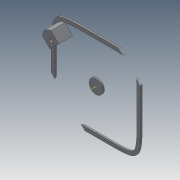
# Autodesk Inventor part: Part1
Saved by Autodesk Inventor 2014 SP1 (Build 180222100, 222)
## iProperties
Created: 2014-04-02
Part Number: Part1
Material: Generic
Document SubType Name: Modeling
Designer: tom
Density: 1 g/cm^3
Appearance: Default
Author: tom
Autodesk Inventor part; units mm, degrees
ref_plane "YZ Plane" through (0, 0, 0) normal (1, 0, 0) x (0, 1, 0)
ref_plane "XZ Plane" through (0, 0, 0) normal (0, 1, 0) x (-1, 0, 0)
ref_plane "XY Plane" through (0, 0, 0) normal (0, 0, 1) x (1, 0, 0)
sketch "Sketch1" plane through (0, 0, 0) normal (0, 0, 1) x (1, 0, 0)
  line L0 (-82.2587, 0) -> (-82.2587, 66.0349) construction
  line L1 (-82.2587, 66.0349) -> (-82.5436, 82.5437) construction
  line L2 (-82.5436, 82.5437) -> (-65.75, 82.0022) construction
  line L3 (-65.75, 82.0022) -> (0.29, 81.9737) construction
  spline S0 degree 4 poles (-82.2587, 0) (-82.2587, 66.0349) (-82.5436, 82.5437) (-65.75, 82.0022) (0.29, 81.9737) knots 1 1 1 1 1 2 2 2 2 2
  spline S1 degree 4 poles (-0.0001, -80.2641) (-66.0349, -80.2631) (-82.5436, -82.5437) (-82.2587, -66.0349) (-82.2587, 0) knots 1 1 1 1 1 2 2 2 2 2
  line L4 (-0.0001, -80.2641) -> (-66.0349, -80.2631) construction
  line L5 (-66.0349, -80.2631) -> (-82.5436, -82.5437) construction
  line L6 (-82.5436, -82.5437) -> (-82.2587, -66.0349) construction
  line L7 (-82.2587, -66.0349) -> (-82.2587, 0) construction
  spline S2 degree 4 poles (81.9738, 0.0005) (81.9826, -66.0349) (82.5437, -82.5436) (66.0349, -80.2652) (-0.0001, -80.2641) knots 1 1 1 1 1 2 2 2 2 2
  line L8 (81.9738, 0.0005) -> (81.9826, -66.0349) construction
  line L9 (81.9826, -66.0349) -> (82.5437, -82.5436) construction
  line L10 (82.5437, -82.5436) -> (66.0349, -80.2652) construction
  line L11 (66.0349, -80.2652) -> (-0.0001, -80.2641) construction
  spline S3 degree 4 poles (0.29, 81.9737) (66.0431, 81.9454) (82.5436, 82.5436) (81.9649, 66.0349) (81.9738, 0.0005) knots 1 1 1 1 1 2 2 2 2 2
  line L12 (0.29, 81.9737) -> (66.0431, 81.9454) construction
  line L13 (66.0431, 81.9454) -> (82.5436, 82.5436) construction
  line L14 (82.5436, 82.5436) -> (81.9649, 66.0349) construction
  line L15 (81.9649, 66.0349) -> (81.9738, 0.0005) construction
  circle A0 centre (0, 0) radius 12.7
  spline S4 degree 5 poles (75.1158, -0.0005) (75.1151, 4.7038) (75.1174, 9.4081) (75.1176, 14.1124) (75.1034, 22.44) (75.0077, 30.7672) (74.9416, 34.3899) (74.7649, 40.6623) (74.3822, 46.9251) (74.1686, 49.5676) (73.6967, 53.9768) (72.8746, 58.3337) (72.4687, 60.0672) (71.6353, 62.8858) (70.347, 65.5172) (69.7572, 66.5071) (68.3459, 68.3278) (66.529, 69.744) (65.543, 70.3346) (62.923, 71.6236) (60.1151, 72.4579) (58.3888, 72.8639) (54.0494, 73.6867) (49.6575, 74.1591) (47.0251, 74.3729) (40.7867, 74.7564) (34.5385, 74.934) (30.9299, 75.0006) (22.6362, 75.0978) (14.342, 75.1137) (9.657, 75.1147) (4.972, 75.1137) (0.287, 75.1157) knots 0 0 0 0 0 0 0.169519 0.169519 0.169519 0.300085 0.300085 0.300085 0.395596 0.395596 0.395596 0.459735 0.459735 0.459735 0.500964 0.500964 0.500964 0.542086 0.542086 0.542086 0.605973 0.605973 0.605973 0.701119 0.701119 0.701119 0.831177 0.831177 0.831177 1 1 1 1 1 1
  spline S5 degree 5 poles (0.287, 75.1157) (-4.4205, 75.1178) (-9.1281, 75.1224) (-13.8357, 75.1248) (-22.1755, 75.114) (-30.5149, 75.0207) (-34.1464, 74.9554) (-40.4414, 74.7792) (-46.7267, 74.3962) (-49.3828, 74.1821) (-53.824, 73.7076) (-58.2129, 72.8821) (-59.9648, 72.4734) (-62.8221, 71.6316) (-65.4927, 70.333) (-66.5029, 69.7357) (-68.3594, 68.3111) (-69.8124, 66.4769) (-70.4194, 65.4828) (-71.7396, 62.8516) (-72.6013, 60.027) (-73.0204, 58.2951) (-73.8722, 53.9442) (-74.3672, 49.5377) (-74.5926, 46.898) (-74.9998, 40.6409) (-75.1937, 34.3731) (-75.2678, 30.7528) (-75.3783, 22.4301) (-75.4, 14.1068) (-75.4022, 9.4045) (-75.4007, 4.7023) (-75.4007, 0) knots 0 0 0 0 0 0 0.168867 0.168867 0.168867 0.299158 0.299158 0.299158 0.394725 0.394725 0.394725 0.459234 0.459234 0.459234 0.50104 0.50104 0.50104 0.542522 0.542522 0.542522 0.606422 0.606422 0.606422 0.701433 0.701433 0.701433 0.831324 0.831324 0.831324 1 1 1 1 1 1
  spline S6 degree 5 poles (-75.4007, 0) (-75.4007, -4.7012) (-75.4022, -9.4023) (-75.4001, -14.1035) (-75.3789, -22.418) (-75.2703, -30.7319) (-75.1974, -34.3444) (-75.0071, -40.5841) (-74.6053, -46.8133) (-74.3834, -49.4328) (-73.8986, -53.7791) (-73.0586, -58.0704) (-72.6483, -59.7625) (-71.8149, -62.4895) (-70.5249, -65.0214) (-69.9429, -65.9585) (-68.5343, -67.6871) (-66.729, -68.9967) (-65.7445, -69.539) (-63.0993, -70.7306) (-60.2841, -71.4698) (-58.5408, -71.8268) (-54.154, -72.5348) (-49.7262, -72.9092) (-47.0698, -73.0702) (-40.7791, -73.3404) (-34.4828, -73.4305) (-30.8476, -73.4541) (-22.4968, -73.4682) (-14.1462, -73.4346) (-9.4308, -73.4169) (-4.7154, -73.406) (0, -73.4061) knots 0 0 0 0 0 0 0.169807 0.169807 0.169807 0.300319 0.300319 0.300319 0.39525 0.39525 0.39525 0.458132 0.458132 0.458132 0.497671 0.497671 0.497671 0.537989 0.537989 0.537989 0.602263 0.602263 0.602263 0.69837 0.69837 0.69837 0.829679 0.829679 0.829679 1 1 1 1 1 1
  spline S7 degree 5 poles (0, -73.4061) (4.7152, -73.4062) (9.4303, -73.4172) (14.1455, -73.435) (22.4946, -73.4688) (30.8439, -73.4549) (34.4778, -73.4313) (40.7693, -73.3414) (47.0553, -73.0712) (49.7083, -72.9103) (54.1262, -72.5365) (58.5029, -71.8289) (60.2396, -71.4725) (63.039, -70.736) (65.6679, -69.5473) (66.6431, -69.0078) (68.4318, -67.7029) (69.8217, -65.9798) (70.395, -65.0454) (71.6681, -62.5142) (72.4851, -59.7907) (72.8873, -58.0982) (73.7081, -53.8036) (74.1766, -49.4561) (74.3898, -46.8349) (74.7726, -40.6019) (74.9483, -34.3591) (75.0139, -30.7448) (75.1085, -22.4272) (75.121, -14.1093) (75.1198, -9.4063) (75.1164, -4.7034) (75.1158, -0.0005) knots 0 0 0 0 0 0 0.170466 0.170466 0.170466 0.301845 0.301845 0.301845 0.397913 0.397913 0.397913 0.462009 0.462009 0.462009 0.502018 0.502018 0.502018 0.541348 0.541348 0.541348 0.604235 0.604235 0.604235 0.699287 0.699287 0.699287 0.829977 0.829977 0.829977 1 1 1 1 1 1
  point P0 (0, 0)
  dimension "d3" = 6.858
  dimension "d0" = 66.04
  dimension "d1" = 66.0349
  dimension "d2" = 82.5487
  dimension "d6" = 25.4
  constraints: 1 centre point, 1 coincident, 24 other
  measures "d0" distance of L3.end L2.end
  measures "d1" distance of L0.start L0.end
  measures "d2" distance from line of L0 L3.end
  measures "d6" diameter of A0
extrude "Extrusion1" add sketch "Sketch1" along normal blind 2.794
sketch "Sketch2" plane through (0, 0, 2.794) normal (0, 0, 1) x (1, 0, 0)
  line L0 (-57.15, 57.15) -> (57.15, 57.15) construction
  line L1 (57.15, 57.15) -> (57.15, -57.15) construction
  line L2 (57.15, -57.15) -> (-57.15, -57.15) construction
  line L3 (-57.15, -57.15) -> (-57.15, 57.15) construction
  circle A0 centre (-57.15, 57.15) radius 3.175
  line L4 (-57.15, 57.15) -> (-50.8638, 50.8638) construction
  line L5 (-50.8638, 50.8638) -> (-42.7816, 58.9461)
  line L6 (-50.8638, 50.8638) -> (-58.9461, 42.7816)
  line L7 (-58.9461, 42.7816) -> (-73.2341, 57.0697)
  line L8 (-42.7816, 58.9461) -> (-56.9328, 73.0973)
  spline S0 degree 5 poles (-75.4007, 0) (-75.4007, 4.7023) (-75.4022, 9.4045) (-75.4, 14.1068) (-75.3783, 22.4301) (-75.2678, 30.7528) (-75.1937, 34.3731) (-74.9998, 40.6409) (-74.5926, 46.898) (-74.3672, 49.5377) (-73.8722, 53.9442) (-73.0204, 58.2951) (-72.6013, 60.027) (-71.7396, 62.8516) (-70.4194, 65.4828) (-69.8124, 66.4769) (-68.3594, 68.3111) (-66.5029, 69.7357) (-65.4927, 70.333) (-62.8221, 71.6316) (-59.9648, 72.4734) (-58.2129, 72.8821) (-53.824, 73.7076) (-49.3828, 74.1821) (-46.7267, 74.3962) (-40.4414, 74.7792) (-34.1464, 74.9554) (-30.5149, 75.0207) (-22.1755, 75.114) (-13.8357, 75.1248) (-9.1281, 75.1224) (-4.4205, 75.1178) (0.287, 75.1157) knots 0 0 0 0 0 0 0.168676 0.168676 0.168676 0.298567 0.298567 0.298567 0.393578 0.393578 0.393578 0.457478 0.457478 0.457478 0.49896 0.49896 0.49896 0.540766 0.540766 0.540766 0.605275 0.605275 0.605275 0.700842 0.700842 0.700842 0.831133 0.831133 0.831133 1 1 1 1 1 1 projected
  point P0 (0, 0)
  dimension "d7" = 114.3
  dimension "d8" = 114.3
  dimension "d9" = 57.15
  dimension "d10" = 57.15
  dimension "d11" = 6.35
  dimension "d12" = 8.89
  dimension "d13" = 11.43
  dimension "d14" = 11.43
  constraints: 18 end point, 3 parallel, 3 perpendicular, 1 centre point, 1 coincident, 1 collinear, 1 horizontal, 3 other
  measures "d7" distance of L1.end L2.end
  measures "d8" distance of L0.end L1.end
  measures "d9" distance from line of point (0, 0) L0
  measures "d10" distance from line of L3 point (0, 0)
  measures "d11" diameter of A0
  measures "d12" distance of L4.start L4.end
  measures "d13" distance of L4.end L5.end
  measures "d14" distance of L4.end L6.end
extrude "Extrusion2" add sketch "Sketch2" along normal blind 25.4
sketch "Sketch3" plane through (0, 0, 2.794) normal (0, 0, -1) x (-1, 0, 0)
  circle A0 centre (57.15, 57.15) radius 3.175 projected
  line L0 (58.9461, 42.7816) -> (42.7816, 58.9461) projected
  line L1 (73.2341, 57.0697) -> (58.9461, 42.7816) projected
  line L2 (42.7816, 58.9461) -> (56.9328, 73.0973) projected
  arc A1 (61.3178, 45.1534) -> (45.1534, 61.3178) centre (57.15, 57.15) ccw
  point P0 (0, 0)
  constraints: 2 point on circle, 2 point on line, 1 centre point, 1 coincident
extrude "Extrusion3" cut sketch "Sketch3" against normal blind 20.32
pattern_circular "Circular Pattern1" count 4 over 360 about axis through (0, 0, 0) along (0, 0, 1) of "Extrusion2", "Extrusion3"
body "Solid1"
